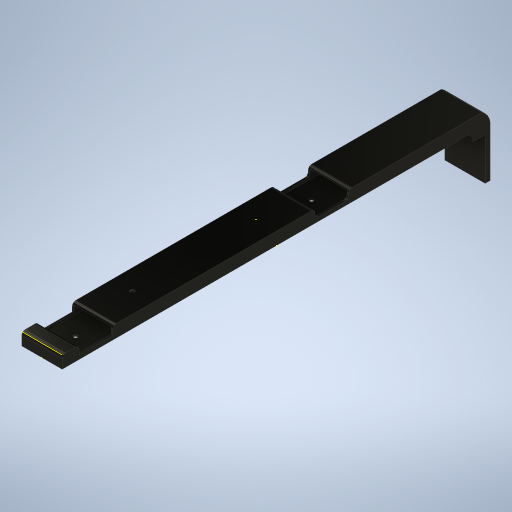
# Autodesk Inventor part: WAFER
Saved by Autodesk Inventor 2023 (Build 270158000, 158)
## iProperties
Created: 2023-10-24
Part Number: WAFER
Material: Generic
Document SubType Name: Modeling
Designer: ASUS
Density: 1 g/cm^3
Appearance: Default
Author: ASUS
Autodesk Inventor part; units mm, degrees
ref_plane "YZ Plane" through (0, 0, 0) normal (1, 0, 0) x (0, 1, 0)
ref_plane "XZ Plane" through (0, 0, 0) normal (0, 1, 0) x (-1, 0, 0)
ref_plane "XY Plane" through (0, 0, 0) normal (0, 0, 1) x (1, 0, 0)
sketch "Sketch1" plane through (0, 0, 0) normal (0, 1, 0) x (-1, 0, 0)
  line L0 (12, 127) -> (-12, 127)
  line L1 (-12, 127) -> (-12, -127)
  line L2 (-12, -127) -> (12, -127)
  line L3 (12, -127) -> (12, 127)
  line L4 (12, 127) -> (-12, -127) construction
  line L5 (-12, 127) -> (12, -127) construction
  point P0 (0, 0)
  dimension "d0" = 24
  dimension "d1" = 254
  constraints: 12 end point, 2 midpoint, 2 parallel, 1 horizontal, 1 perpendicular
  measures "d0" distance of L2.end L1.end
  measures "d1" distance of L1.end L0.end
extrude "Extrusion1" add sketch "Sketch1" along normal blind 7.4
sketch "Sketch2" plane through (-12, 0, 127) normal (0, 0, 1) x (1, 0, 0)
  line L0 (0, 7.4) -> (24, 7.4) projected
  line L1 (24, 0) -> (24, 7.4) projected
  line L2 (0, 7.4) -> (24, 7.4)
  line L3 (24, 7.4) -> (24, 0)
  line L4 (24, 0) -> (0, 0)
  line L5 (0, 0) -> (0, 7.4)
  line L6 (0, 7.4) -> (24, 0) construction
  line L7 (24, 7.4) -> (0, 0) construction
  line L8 (1, 1) -> (23, 1)
  line L9 (23, 1) -> (23, 6.4)
  line L10 (23, 6.4) -> (1, 6.4)
  line L11 (1, 6.4) -> (1, 1)
  point P0 (12, 0)
  point P1 (12, 3.7)
  dimension "d4" = 1
  constraints: 20 end point, 4 parallel, 2 midpoint, 2 perpendicular, 1 horizontal, 3 other
  measures "d4" distance between parallel lines of L4 L8
extrude "Extrusion2" cut sketch "Sketch2" against normal blind 248 contours L11 L10 L9 L8
sketch "Sketch3" plane through (0, 0, 0) normal (0, -1, 0) x (1, 0, 0)
  line L0 (-12, -127) -> (12, -127)
  line L1 (12, -127) -> (-12, -127) projected
  line L2 (-12, -127) -> (-12, -112)
  line L3 (12, -127) -> (12, -117)
  line L4 (12, 127) -> (12, -127) projected
  line L5 (12, -117) -> (-12, -117)
  line L6 (-12, -127) -> (-12, 127) projected
  point P0 (0, 0)
  dimension "d8" = 10
  constraints: 8 end point, 2 perpendicular, 2 point on line
  measures "d8" distance of L0.end L3.end
extrude "Extrusion3" add sketch "Sketch3" along normal blind 30
sketch "Sketch4" plane through (0, -30, 0) normal (0, -1, 0) x (1, 0, 0)
  line L0 (-12, -117) -> (12, -117) projected
  line L1 (-12, -127) -> (-12, 127) projected
  line L2 (12, -117) -> (-12, -117)
  line L3 (-12, -117) -> (-12, -127)
  line L4 (-12, -127) -> (12, -127)
  line L5 (12, -127) -> (12, -117)
  line L6 (10.5, -118.5) -> (-10.5, -118.5)
  line L7 (-10.5, -118.5) -> (-10.5, -125.5)
  line L8 (-10.5, -125.5) -> (10.5, -125.5)
  line L9 (10.5, -125.5) -> (10.5, -118.5)
  point P0 (0, 0)
  dimension "d11" = 1.5
  constraints: 16 end point, 4 parallel, 2 perpendicular, 1 horizontal, 3 other
  measures "d11" distance between parallel lines of L5 L9
extrude "Extrusion4" cut sketch "Sketch4" against normal blind 36 contours L9 L8 L7 L6
fillet "Fillet2" radius 5 1 edges at (0, 0, -117)
sketch "Sketch6" plane through (-12, 0, 127) normal (-1, 0, 0) x (0, 0, 1)
  line L0 (-254, -30) -> (-254, 7.4) projected
  line L1 (-254, 7.4) -> (-254, 3.9)
  line L2 (-254, 3.9) -> (-254, 2.4)
  line L3 (-254, -30) -> (-254, 7.4) projected
  line L4 (-254, 7.4) -> (0, 7.4) projected
  line L5 (-254, 2.4) -> (-254, -0.6)
  line L6 (-254, 7.4) -> (-249, 7.4)
  arc A0 (-249, 7.4) -> (-254, -0.6) centre (-244.0227, -1.2733) ccw
  point P0 (-127, 0)
  dimension "d21" = 3.5
  dimension "d23" = 1.5
  dimension "d26" = 3
  dimension "d27" = 5
  dimension "d28" = 10
  constraints: 8 end point, 4 point on line, 2 point on circle, 1 centre point
  measures "d21" distance of L0.end L1.end
  measures "d23" distance of L1.end L2.end
  measures "d26" distance of L2.end L5.end
  measures "d27" distance of L0.end L6.end
  measures "d28" radius of A0
extrude "Extrusion6" cut sketch "Sketch6" against normal blind 36
sketch "Sketch7" plane through (0, 7.4, 0) normal (0, 1, 0) x (1, 0, 0)
  line L0 (-12, -127) -> (12, -127) projected
  point P0 (0, 0)
sketch "Sketch8" plane through (-12, 0, 127) normal (-1, 0, 0) x (0, 0, 1)
  line L0 (0, 7.4) -> (-20, 7.4)
  line L1 (0, 7.4) -> (-249, 7.4) projected
  line L2 (0, 7.4) -> (0, 3.7)
  line L3 (-20, 3.7) -> (-30, 3.7)
  line L4 (-30, 3.7) -> (-30, 7.4)
  line L5 (-249, 7.4) -> (0, 7.4) projected
  line L6 (-30, 7.4) -> (-10, 7.4)
  line L7 (-10, 7.4) -> (-10, 3.7)
  line L8 (-20, 3.7) -> (-10, 3.7)
  line L9 (-30, 7.4) -> (-10, 7.4)
  point P0 (-127, 0)
  dimension "d32" = 20
  dimension "d33" = 3.7
  dimension "d34" = 10
  dimension "d35" = 20
  constraints: 16 end point, 3 point on line, 2 horizontal, 1 collinear, 1 vertical
  measures "d32" distance of L0.start L0.end
  measures "d33" distance of L0.end L3.start
  measures "d34" distance of L3.start L3.end
  measures "d35" distance of L4.end L6.end
extrude "Extrusion7" cut sketch "Sketch8" against normal blind 30
sketch "Sketch9" plane through (-12, 0, 127) normal (0, 0, 1) x (1, 0, 0)
  point P0 (12, 0)
sketch "Sketch10" plane through (-12, 0, 127) normal (0, 0, 1) x (1, 0, 0)
  line L0 (23, 6.4) -> (23, 1) projected
  line L1 (1, 6.4) -> (23, 6.4)
  line L2 (23, 6.4) -> (23, 1)
  line L3 (23, 1) -> (1, 1)
  line L4 (1, 1) -> (1, 6.4)
  point P0 (12, 0)
  constraints: 8 end point, 2 parallel, 1 horizontal, 1 perpendicular
extrude "Extrusion8" add sketch "Sketch10" against normal blind 10
sketch "Sketch11" plane through (-10.5, 1, -118.5) normal (0, 1, 0) x (1, 0, 0)
  line L0 (-0.5, -235.5) -> (21.5, -235.5) projected
  line L1 (21.5, -235.5) -> (10.5, -235.5)
  circle A0 centre (10.5, -225.5) radius 1.25
  point P0 (10.5, -118.5)
  dimension "d40" = 11
  dimension "d42" = 2.5
  constraints: 2 end point, 1 centre point, 1 midpoint
  measures "d40" distance of L0.end L1.end
  measures "d42" diameter of A0
extrude "Extrusion9" cut sketch "Sketch11" against normal blind 10
thread "Thread1" size "M2.5x0.45" class "6H" standard "ANSI Metric M Profile" full length
sketch "Sketch12" plane through (0, 7.4, 0) normal (0, 1, 0) x (1, 0, 0)
  line L0 (-12, -97) -> (12, -97) projected
  circle A0 centre (0, -73.3) radius 1.25
  point P0 (0, 0)
  dimension "d48" = 2.5
  constraints: 1 centre point
  measures "d48" diameter of A0
extrude "Extrusion10" cut sketch "Sketch12" against normal blind 5
thread "Thread2" size "M2.5x0.45" class "6H" standard "ANSI Metric M Profile" full length
sketch "Sketch13" plane through (12, 0, 127) normal (1, 0, 0) x (0, 0, -1)
  line L0 (254, -30) -> (244, -30) projected
  line L1 (254, -30) -> (252.5, -30)
  line L2 (252.5, -30) -> (252.5, -5)
  line L3 (252.5, -5) -> (244, -5)
  line L4 (244, -5) -> (244, -30)
  line L5 (244, -30) -> (252.5, -30)
  point P0 (127, 0)
  dimension "d53" = 1.5
  dimension "d54" = 25
  constraints: 10 end point, 3 perpendicular, 1 horizontal, 1 point on line
  measures "d53" distance of L0.start L1.end
  measures "d54" distance of L1.end L2.end
extrude "Extrusion11" cut sketch "Sketch13" against normal blind 100
sketch "Sketch14" plane through (0, 7.4, 0) normal (0, 1, 0) x (1, 0, 0)
  point P0 (0, 0)
fillet "Fillet4" radius 2 1 edges at (0, 1, 117)
fillet "Fillet5" radius 2 1 edges at (0, 7.4, 117)
fillet "Fillet6" radius 2 1 edges at (0, 7.4, 97)
fillet "Fillet7" radius 2 1 edges at (0, 7.4, 127)
sketch "Sketch17" plane through (0, 7.4, 0) normal (0, 1, 0) x (1, 0, 0)
  point P0 (0, 0)
sketch "Sketch18" plane through (-12, -30, -125.5) normal (0, 0, 1) x (1, 0, 0)
  line L0 (0, 0) -> (24, 0) projected
  line L1 (0, 0) -> (24, 0)
  line L2 (24, 25) -> (22.5, 25) projected
  line L3 (24, 0) -> (24, 25)
  line L4 (24, 25) -> (22.5, 25)
  line L5 (22.5, 25) -> (22.5, 29.5155)
  line L6 (22.5, 25) -> (22.5, 34.031) projected
  line L7 (22.5, 29.5155) -> (1.5, 29.5155)
  line L8 (1.5, 25) -> (1.5, 34.031) projected
  line L9 (1.5, 29.5155) -> (1.5, 25)
  line L10 (1.5, 25) -> (0, 25)
  line L11 (0, 25) -> (0, 0)
  point P0 (12, 30)
  constraints: 16 end point, 2 collinear, 2 midpoint, 2 perpendicular, 1 horizontal, 1 vertical
extrude "Extrusion14" add sketch "Sketch18" along normal blind 1.5
sketch "Sketch19" plane through (12, -30, -127) normal (0, 0, -1) x (-1, 0, 0)
  point P0 (12, 30)
sketch "Sketch20" plane through (-12, -30, -124) normal (0, 0, 1) x (1, 0, 0)
  point P0 (12, 30)
sketch "Sketch21" plane through (12, -30, -127) normal (0, 0, -1) x (-1, 0, 0)
  line L0 (24, 0) -> (0, 0) projected
  circle A0 centre (12, 25) radius 1.45
  point P0 (12, 30)
  dimension "d83" = 2.9
  constraints: 1 centre point
  measures "d83" diameter of A0
extrude "Extrusion15" cut sketch "Sketch21" against normal blind 4
thread "Thread4" size "M3x0.5" class "6H" standard "ANSI Metric M Profile" full length
sketch "Sketch22" plane through (12, 0, 127) normal (1, 0, 0) x (0, 0, -1)
  line L0 (170, 2.5) -> (150, 2.5)
  line L1 (150, 2.5) -> (150, 7.4)
  line L2 (32, 7.4) -> (249, 7.4) projected
  line L3 (170, 2.5) -> (170, 7.4)
  line L4 (150, 7.4) -> (170, 7.4)
  point P0 (127, 0)
  point P1 (0, 0)
  dimension "d91" = 20
  constraints: 8 end point, 2 perpendicular, 2 point on line, 1 vertical
  measures "d91" distance of L0.start L0.end
extrude "Extrusion16" cut sketch "Sketch22" against normal blind 25
sketch "Sketch23" plane through (12, 0, 127) normal (1, 0, 0) x (0, 0, -1)
  line L0 (10, 3.7) -> (30, 3.7) projected
  line L1 (0, 0) -> (239, 0) projected
  line L2 (10, 3) -> (10, 3.7) projected
  line L3 (10, 2.5) -> (10, 3.7)
  line L4 (10, 2.5) -> (30, 2.5)
  line L5 (30, 2.5) -> (30, 3.7)
  line L6 (30, 3.7) -> (30, 5.4) projected
  line L7 (10, 3.7) -> (30, 3.7)
  point P0 (127, 0)
  constraints: 8 end point, 1 horizontal, 1 parallel, 1 perpendicular
extrude "Extrusion17" cut sketch "Sketch23" against normal blind 25
fillet "Fillet8" radius 2 6 edges at (0, 7.4, -23) (11.5, 2.5, -23) (-11.5, 2.5, -23) (11.5, 2.5, -43) (-11.5, 2.5, -43) (0, 7.4, -43)
sketch "Sketch24" plane through (12, 0, 127) normal (1, 0, 0) x (0, 0, -1)
  point P0 (127, 0)
sketch "Sketch25" plane through (-10.5, 1, -118.5) normal (0, 1, 0) x (1, 0, 0)
  line L0 (-0.5, -77.5) -> (-0.5, -93.5) projected
  line L1 (21.5, -233.5) -> (21.5, 2.5) projected
  circle A0 centre (10.5, -85.5) radius 1.25
  point P0 (10.5, -118.5)
  dimension "d99" = 2.5
  constraints: 1 centre point
  measures "d99" diameter of A0
extrude "Extrusion18" cut sketch "Sketch25" against normal blind 25
sketch "Sketch26" plane through (12, 0, 127) normal (1, 0, 0) x (0, 0, -1)
  point P0 (127, 0)
body "Solid1"
